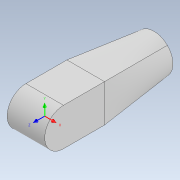
# Autodesk Inventor part: shank
Saved by Autodesk Inventor 2020 (Build 240168000, 168)
## iProperties
Created: 2021-01-29
Part Number: shank
Material: Generic
Document SubType Name: Modeling
Designer: DELL
Density: 1 g/cm^3
Appearance: Default
Author: DELL
Autodesk Inventor part; units mm, degrees
ref_plane "YZ Plane" through (0, 0, 0) normal (1, 0, 0) x (0, 1, 0)
ref_plane "XZ Plane" through (0, 0, 0) normal (0, 1, 0) x (-1, 0, 0)
sketch "Sketch1" plane through (0, 0, 0) normal (1, 0, 0) x (0, 1, 0)
  circle A0 centre (0, 0) radius 27.5
  line L0 (-27.5, 0) -> (-27.5, -60)
  line L1 (-27.5, -60) -> (27.5, -60)
  line L2 (27.5, -60) -> (27.5, 0)
  dimension "d0" = 55
  dimension "d1" = 60
  constraints: 6 end point, 2 perpendicular, 2 point on circle, 2 tangent, 1 centre point, 1 coincident, 1 vertical
  measures "d0" diameter of A0
  measures "d1" distance from line of point (0, 0) L1
extrude "Extrusion1" add sketch "Sketch1" along normal mid plane 55
sketch "Sketch2" plane through (27.5, 27.5, -60) normal (0, 0, -1) x (-1, 0, 0)
  line L0 (0, -55) -> (0, 0) projected
  line L1 (55, 0) -> (0, 0)
  line L2 (0, 0) -> (0, -55)
  line L3 (0, -55) -> (55, -55)
  line L4 (55, -55) -> (55, 0)
  line L5 (55, 0) -> (0, -55) construction
  line L6 (0, 0) -> (55, -55) construction
  point P0 (27.5, -27.5)
  constraints: 12 end point, 2 midpoint, 2 parallel, 1 horizontal, 1 perpendicular
ref_plane "Work Plane1" through (27.5, 27.5, -160) normal (0, 0, -1) x (-1, 0, 0)
sketch "Sketch3" plane through (27.5, 27.5, -160) normal (0, 0, -1) x (-1, 0, 0)
  circle A0 centre (27.5, -27.5) radius 27.5
  line L0 (55, -55) -> (0, -55) projected
  point P0 (27.5, -27.5)
  constraints: 1 centre point, 1 coincident, 1 tangent
loft "Loft1" add profiles "Sketch2", "Sketch3"
sketch "Sketch4" plane through (27.5, 27.5, -160) normal (0, 0, -1) x (-1, 0, 0)
  circle A0 centre (27.5, -27.5) radius 15
  point P0 (27.5, -27.5)
  dimension "d9" = 30
  constraints: 1 centre point, 1 coincident
  measures "d9" diameter of A0
extrude "Extrusion2" cut sketch "Sketch4" against normal blind 60
body "Solid1"
